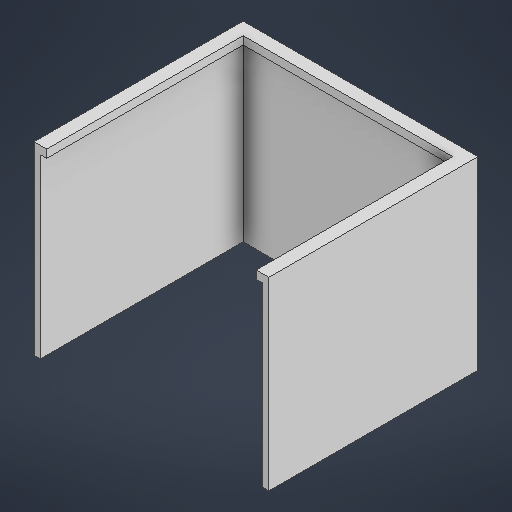
# Autodesk Inventor part: Cylinder Galvo Housing
Saved by Autodesk Inventor 2025 (Build 290162000, 162)
## iProperties
Created: 2024-06-10
Part Number: Cylinder Galvo Housing
Material: Generic
Document SubType Name: Modeling
Designer: mayhe
Density: 1 g/cm^3
Appearance: Default
Author: mayhe
Autodesk Inventor part; units mm, degrees
ref_plane "YZ Plane" through (0, 0, 0) normal (1, 0, 0) x (0, 1, 0)
ref_plane "XZ Plane" through (0, 0, 0) normal (0, 1, 0) x (-1, 0, 0)
ref_plane "XY Plane" through (0, 0, 0) normal (0, 0, 1) x (1, 0, 0)
sketch "Sketch1" plane through (0, 0, 0) normal (0, 1, 0) x (-1, 0, 0)
  line L0 (-73, 65) -> (73, 65)
  line L1 (73, 65) -> (73, -65)
  line L2 (73, -65) -> (-73, -65)
  line L3 (-73, -65) -> (-73, 65)
  line L4 (-73, 65) -> (73, -65) construction
  line L5 (73, 65) -> (-73, -65) construction
  point P0 (0, 0)
  dimension "d0" = 146
  dimension "d1" = 130
  constraints: 12 end point, 2 midpoint, 2 parallel, 1 horizontal, 1 perpendicular
  measures "d0" distance of L1.end L2.end
  measures "d1" distance of L0.end L1.end
extrude "Extrusion1" add sketch "Sketch1" along normal blind 115
sketch "Sketch2" plane through (0, 0, 0) normal (0, -1, 0) x (1, 0, 0)
  line L0 (-69.125, -61.125) -> (69.125, -61.125)
  line L1 (69.125, -61.125) -> (69.125, 61.125)
  line L2 (69.125, 61.125) -> (-69.125, 61.125)
  line L3 (-69.125, 61.125) -> (-69.125, -61.125)
  line L4 (-69.125, -61.125) -> (69.125, 61.125) construction
  line L5 (69.125, -61.125) -> (-69.125, 61.125) construction
  line L6 (-69.125, 61.125) -> (69.125, 61.125)
  line L7 (69.125, 61.125) -> (69.125, 91.125)
  line L8 (69.125, 91.125) -> (-69.125, 91.125)
  line L9 (-69.125, 91.125) -> (-69.125, 61.125)
  point P0 (0, 0)
  dimension "d4" = 138.25
  dimension "d5" = 122.25
  dimension "d6" = 138.25
  dimension "d7" = 30
  constraints: 20 end point, 4 parallel, 2 horizontal, 2 midpoint, 2 perpendicular
  measures "d4" distance of L2.end L1.end
  measures "d5" distance of L1.end L0.end
  measures "d6" distance of L8.end L7.end
  measures "d7" distance of L7.end L6.end
extrude "Extrusion2" cut sketch "Sketch2" against normal through all
sketch "Sketch3" plane through (0, 115, 0) normal (0, 1, 0) x (1, 0, 0)
  line L0 (-69.125, 61.125) -> (69.125, 61.125) projected
  line L1 (69.125, 61.125) -> (69.125, -65) projected
  line L2 (-69.125, 61.125) -> (69.125, 61.125)
  line L3 (69.125, 61.125) -> (69.125, -65)
  line L4 (69.125, -65) -> (-69.125, -65)
  line L5 (-69.125, -65) -> (-69.125, 61.125)
  line L6 (-65.125, -57.125) -> (65.125, -57.125)
  line L7 (65.125, -57.125) -> (65.125, 57.125)
  line L8 (65.125, 57.125) -> (-65.125, 57.125)
  line L9 (-65.125, 57.125) -> (-65.125, -57.125)
  line L10 (-65.125, -57.125) -> (65.125, 57.125) construction
  line L11 (65.125, -57.125) -> (-65.125, 57.125) construction
  line L12 (65.125, -57.125) -> (65.125, -65)
  line L13 (-65.125, -57.125) -> (-65.125, -65)
  point P0 (0, 0)
  dimension "d10" = 4
  dimension "d11" = 4
  constraints: 24 end point, 4 parallel, 4 perpendicular, 2 horizontal, 2 midpoint, 2 point on line
  measures "d10" distance between parallel lines of L9 L5
  measures "d11" distance between parallel lines of L0 L8
extrude "Extrusion3" add sketch "Sketch3" against normal blind 5 contours L0 L1 L4 L12 L7 L8 L9 L13 L5
body "Solid1"
